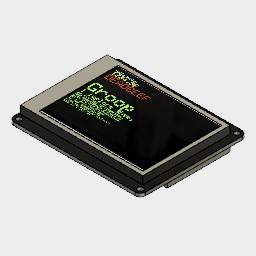
3315  2.4 TFT Feather Wing (Autodesk Fusion 360 design; units mm, degrees)
Autodesk Fusion 360 part; units mm, degrees
note: some values were not read from the file. Set by a fixed rule: which sketch regions a step uses.
sketch "pcb" plane through (0, 0, 0) normal (0, 0, 1) x (1, 0, 0)
  line L0 (0, 0) -> (64.77, 0)
  line L1 (64.77, 0) -> (64.77, 52.578)
  line L2 (64.77, 52.578) -> (0, 52.578)
  line L3 (0, 52.578) -> (0, 0)
  circle A0 centre (2.54, 50.038) radius 1.27
  line L4 (32.385, 52.578) -> (32.385, 0) construction
  line L5 (0, 26.289) -> (64.77, 26.289) construction
  circle A1 centre (62.23, 50.038) radius 1.27
  circle A2 centre (2.54, 2.54) radius 1.27
  circle A3 centre (62.23, 2.54) radius 1.27
  dimension "d1" = 64.77
  dimension "d2" = 52.578
  dimension "d3" = 2.54
  dimension "d4" = 2.54
  dimension "d5" = 2.54
  measures "d1" distance of L1.end L2.end
  measures "d2" distance of L0.start L2.end
  measures "d3" diameter of A0
  measures "d4" distance of L3 A0.centre
  measures "d5" distance of L2 A0.centre
extrude "Extrude1" add sketch "pcb" along normal blind 1.6 makes body 1
fillet "Fillet1" radius 2.54 4 edges at (64.77, 0, 0.8) (0, 0, 0.8) (0, 52.578, 0.8) (64.77, 52.578, 0.8) on bodies 1
sketch "bottom" plane through (0, 0, 0) normal (0, 0, -1) x (1, 0, 0)
  circle A0 centre (62.23, -50.038) radius 1.27
  circle A1 centre (2.54, -2.54) radius 1.27
  circle A2 centre (62.23, -2.54) radius 1.27
  circle A3 centre (2.54, -50.038) radius 1.27
  arc A4 (62.23, -52.578) -> (64.77, -50.038) centre (62.23, -50.038) ccw
  line L0 (64.77, -50.038) -> (64.77, -2.54)
  arc A5 (64.77, -2.54) -> (62.23, 0) centre (62.23, -2.54) ccw
  line L1 (62.23, 0) -> (2.54, 0)
  arc A6 (2.54, 0) -> (0, -2.54) centre (2.54, -2.54) ccw
  line L2 (0, -2.54) -> (0, -50.038)
  arc A7 (0, -50.038) -> (2.54, -52.578) centre (2.54, -50.038) ccw
  line L3 (2.54, -52.578) -> (62.23, -52.578)
  line L4 (62.97, -45.978) -> (57.97, -45.978)
  line L5 (57.97, -45.978) -> (57.97, -14.978)
  line L6 (57.97, -14.978) -> (62.97, -14.978)
  line L7 (62.97, -14.978) -> (62.97, -45.978)
  line L8 (40.17, -45.978) -> (35.17, -45.978)
  line L9 (35.17, -45.978) -> (35.17, -4.978)
  line L10 (35.17, -4.978) -> (40.17, -4.978)
  line L11 (40.17, -4.978) -> (40.17, -45.978)
  line L12 (1.6, -6.8) -> (7.6, -6.8)
  line L13 (7.6, -6.8) -> (7.6, -12.8)
  line L14 (7.6, -12.8) -> (1.6, -12.8)
  line L15 (1.6, -12.8) -> (1.6, -6.8)
  line L16 (1.6, -6.8) -> (7.6, -12.8) construction
  line L17 (7.6, -6.8) -> (1.6, -12.8) construction
  circle A8 centre (4.6, -9.8) radius 1.5
  line L18 (5.5, -17.4) -> (2, -17.4)
  line L19 (2, -17.4) -> (2, -24.4)
  line L20 (2, -24.4) -> (5.5, -24.4)
  line L21 (5.5, -24.4) -> (5.5, -17.4)
  line L22 (15.5, -43.978) -> (0, -43.978)
  line L23 (0, -43.978) -> (0, -29.978)
  line L24 (0, -29.978) -> (15.5, -29.978)
  line L25 (15.5, -29.978) -> (15.5, -43.978)
  point P0 (4.6, -9.8)
  dimension "d9" = 5
  dimension "d10" = 5
  dimension "d11" = 31
  dimension "d12" = 41
  dimension "d13" = 6.6
  dimension "d14" = 6.6
  dimension "d15" = 1.8
  dimension "d16" = 17.8
  dimension "d19" = 6
  dimension "d20" = 6
  dimension "d21" = 6.8
  dimension "d22" = 1.6
  dimension "d23" = 3
  dimension "d28" = 3.5
  dimension "d29" = 7
  dimension "d30" = 2
  dimension "d31" = 17.4
  dimension "d32" = 15.5
  dimension "d33" = 14
  dimension "d34" = 8.6
  measures "d9" distance of L5.end L6.end
  measures "d10" distance of L9.end L10.end
  measures "d11" distance of L4.start L6.end
  measures "d12" distance of L8.start L10.end
  measures "d13" distance of L3 L4
  measures "d14" distance of L3 L8
  measures "d15" distance of L0 L7
  measures "d16" distance of L5 L11
  measures "d19" distance of L13.end L14.end
  measures "d20" distance of L12.end L13.end
  measures "d21" distance of L1 L12
  measures "d22" distance of L2 L15
  measures "d23" diameter of A8
  measures "d28" distance of L18.start L18.end
  measures "d29" distance of L18.start L20.end
  measures "d30" distance of L2 L19
  measures "d31" distance of L1 L18
  measures "d32" distance of L22.start L22.end
  measures "d33" distance of L22.start L24.end
  measures "d34" distance of L3 L22
extrude "Extrude2" add sketch "bottom" along normal blind 3.9 separate body contours L4 L5 L6 L7 | L8 L9 L10 L11 makes body 2 at (61.3033, 25.3113, 0) makes body 3 at (38.5033, 32.3113, 0)
extrude "Extrude3" add sketch "bottom" along normal blind 1.8 separate body contours L12 L13 L14 L15 | A8 makes body 4
extrude "Extrude4" add sketch "bottom" along normal blind 3 separate body contours A8 makes body 5
extrude "Extrude5" add sketch "bottom" along normal blind 1.4 separate body contours L18 L19 L20 L21 makes body 6
extrude "Extrude6" add sketch "bottom" along normal blind 1.7 separate body contours L2 L22 L23 L24 L25 makes body 7
sketch "microSD" plane through (0, 0, -1.7) normal (0, 0, -1) x (1, 0, 0)
  line L0 (15.5, -29.978) -> (0, -29.978)
  line L1 (0, -29.978) -> (0, -43.978)
  line L2 (0, -43.978) -> (15.5, -43.978)
  line L3 (15.5, -43.978) -> (15.5, -29.978)
  circle A0 centre (-8.5, -35.5) radius 11
  dimension "d39" = 22
  measures "d39" diameter of A0
extrude "Extrude7" cut sketch "microSD" against normal blind 1.7 contours L0 L1 A0 picked at (0.2923, -37.9037) bodies 7
sketch "switch" plane through (0, 0, -1.4) normal (0, 0, -1) x (1, 0, 0)
  line L0 (5.5, -24.4) -> (5.5, -17.4)
  line L1 (5.5, -17.4) -> (2, -17.4)
  line L2 (2, -17.4) -> (2, -24.4)
  line L3 (2, -24.4) -> (5.5, -24.4)
  line L4 (2, -20.9) -> (5.5, -20.9)
  line L5 (2, -19.4) -> (3, -19.4)
  line L6 (3, -19.4) -> (3, -22.4)
  line L7 (3, -22.4) -> (2, -22.4)
  line L8 (2, -22.4) -> (2, -19.4)
  line L9 (3, -20.9) -> (2, -20.9) construction
  dimension "d42" = 3
  dimension "d43" = 1
  measures "d42" distance of L5.end L6.end
  measures "d43" distance of L6.end L7.end
extrude "Extrude8" add sketch "switch" along normal blind 1 separate body contours L2 L4 L6 L7 L8 makes body 8
sketch "display" plane through (0, 0, 1.6) normal (0, 0, 1) x (-1, 0, 0)
  arc A0 (-64.77, -50.038) -> (-62.23, -52.578) centre (-62.23, -50.038) ccw
  line L0 (-62.23, -52.578) -> (-2.54, -52.578)
  arc A1 (-2.54, -52.578) -> (0, -50.038) centre (-2.54, -50.038) ccw
  line L1 (0, -50.038) -> (0, -2.54)
  arc A2 (0, -2.54) -> (-2.54, 0) centre (-2.54, -2.54) ccw
  line L2 (-2.54, 0) -> (-62.23, 0)
  arc A3 (-62.23, 0) -> (-64.77, -2.54) centre (-62.23, -2.54) ccw
  line L3 (-64.77, -2.54) -> (-64.77, -50.038)
  circle A4 centre (-62.23, -50.038) radius 1.27
  circle A5 centre (-2.54, -2.54) radius 1.27
  circle A6 centre (-62.23, -2.54) radius 1.27
  circle A7 centre (-2.54, -50.038) radius 1.27
  line L4 (-0.8, -47.778) -> (-61, -47.778)
  line L5 (-61, -47.778) -> (-61, -4.978)
  line L6 (-61, -4.978) -> (-0.8, -4.978)
  line L7 (-0.8, -4.978) -> (-0.8, -47.778)
  dimension "d46" = 60.2
  dimension "d47" = 42.8
  dimension "d48" = 4.8
  dimension "d49" = 0.8
  measures "d46" distance of L4.start L4.end
  measures "d47" distance of L4.start L6.end
  measures "d48" distance of L0 L4
  measures "d49" distance of L1 L7
extrude "Extrude9" add sketch "display" along normal blind 3.9 separate body contours L4 L5 L6 L7 makes body 9
sketch "view" plane through (0, 0, 5.5) normal (0, 0, 1) x (-1, 0, 0)
  line L0 (-0.8, -4.978) -> (-61, -4.978)
  line L1 (-61, -4.978) -> (-61, -47.778)
  line L2 (-61, -47.778) -> (-0.8, -47.778)
  line L3 (-0.8, -47.778) -> (-0.8, -4.978)
  line L4 (-8, -45.778) -> (-59, -45.778)
  line L5 (-59, -45.778) -> (-59, -6.978)
  line L6 (-59, -6.978) -> (-8, -6.978)
  line L7 (-8, -6.978) -> (-8, -45.778)
  dimension "d52" = 2
  dimension "d53" = 2
  dimension "d54" = 2
  dimension "d55" = 7.2
  measures "d52" distance of L0 L6
  measures "d53" distance of L1 L5
  measures "d54" distance of L2 L4
  measures "d55" distance of L3 L7
extrude "Extrude10" cut sketch "view" against normal blind 0.2 contours L4 L5 L6 L7 bodies 9
ref_plane "WorkPlane1" through (30.9, 26.378, 5.7) normal (0, 0, 1) x (1, 0, 0) in component "mount"
sketch "Sketch1" plane through (30.9, 26.378, 5.7) normal (0, 0, 1) x (1, 0, 0) in component "mount"
  line L0 (-32.9, 28.2) -> (35.87, 28.2)
  line L1 (35.87, 28.2) -> (35.87, -28.378)
  line L2 (35.87, -28.378) -> (-32.9, -28.378)
  line L3 (-32.9, -28.378) -> (-32.9, 28.2)
  line L4 (31.33, 26.2) -> (-28.36, 26.2) construction
  line L5 (33.87, -23.838) -> (33.87, 23.66) construction
  line L6 (-30.9, 23.66) -> (-30.9, -23.838) construction
  line L7 (-28.36, -26.378) -> (31.33, -26.378) construction
  line L8 (-22.9, -19.4) -> (28.1, -19.4)
  line L9 (28.1, -19.4) -> (28.1, 19.4)
  line L10 (28.1, 19.4) -> (-22.9, 19.4)
  line L11 (-22.9, 19.4) -> (-22.9, -19.4)
  circle A0 centre (-28.36, -23.838) radius 1.27
  circle A1 centre (31.33, -23.838) radius 1.27
  circle A2 centre (31.33, 23.66) radius 1.27
  circle A3 centre (-28.36, 23.66) radius 1.27
  line L12 (30.1, -21.4) -> (-30.1, -21.4) construction
  line L13 (-30.1, -21.4) -> (-30.1, 21.4) construction
  line L14 (-30.1, 21.4) -> (30.1, 21.4) construction
  line L15 (30.1, 21.4) -> (30.1, -21.4) construction
  circle A4 centre (-28.36, -23.838) radius 2.77
  circle A5 centre (31.33, 23.66) radius 2.77
  circle A6 centre (-28.36, 23.66) radius 2.77
  line L16 (-30.7, -22) -> (-30.7, 22)
  line L17 (-30.7, 22) -> (30.7, 22)
  line L18 (30.7, 22) -> (30.7, -22)
  line L19 (30.7, -22) -> (-30.7, -22)
  circle A7 centre (31.33, -23.838) radius 2.77
  point P0 (30.06, -23.838)
  dimension "d59" = 2
  dimension "d60" = 2
  dimension "d61" = 2
  dimension "d62" = 2
  dimension "d65" = 1.5
  dimension "d66" = 1.5
  dimension "d67" = 1.5
  dimension "d68" = 1.5
  dimension "d74" = 0.6
  measures "d59" distance of L0 L4
  measures "d60" distance of L1 L5
  measures "d61" distance of L3 L6
  measures "d62" distance of L2 L7
extrude "Extrude1'" add sketch "Sketch1" along normal blind 1 separate body contours L0 L1 L2 L3 | A0 | A1 | A2 | A3 | A4 L19 | A4 L19 | A4 A5 A6 L16 L17 L18 L19 A7 | L18 L19 A7 | L18 L19 A7 | A5 L17 L18 | A5 L17 L18 | A6 L17 | A6 L17 makes body 10 in component "mount"
extrude "Extrude2'" add sketch "Sketch1" against normal up to surface (4.1 mm away) contours A0 | A1 | A2 | A3 | A4 L19 | A4 L19 | L18 L19 A7 | L18 L19 A7 | A5 L17 L18 | A5 L17 L18 | A6 L17 | A6 L17 bodies 10 in component "mount"
extrude "Extrude3'" add sketch "Sketch1" against normal blind 6.5 contours A0 | A1 | A2 | A3 bodies 10 in component "mount"
fillet "Fillet1'" radius 2.54 4 edges at (-2, -2, 6.2) (66.77, -2, 6.2) (-2, 54.578, 6.2) (66.77, 54.578, 6.2) on bodies 10 in component "mount"
extrude "Extrude4'" cut sketch "Sketch1" against normal blind 5 contours A4 L19 | A4 A5 A6 L16 L17 L18 L19 A7 | L18 L19 A7 | A5 L17 L18 | A6 L17 picked at (-28.2304, -21.6985) picked at (30.5911, -21.4597) picked at (30.5768, 21.3464) picked at (-27.9175, 21.7429) bodies 10 in component "mount"
sketch "32 holes" plane through (0, 0, -3.9) normal (0, 0, -1) x (1, 0, 0)
  line L0 (40.17, -4.978) -> (35.17, -4.978)
  line L1 (35.17, -4.978) -> (35.17, -45.978)
  line L2 (35.17, -45.978) -> (40.17, -45.978)
  line L3 (40.17, -45.978) -> (40.17, -4.978)
  line L4 (37.67, -4.978) -> (37.67, -45.978) construction
  line L5 (38.94, -45.978) -> (38.94, -4.978) construction
  circle A0 centre (38.94, -44.708) radius 0.635
  circle A1 centre (38.94, -42.168) radius 0.635
  circle A2 centre (38.94, -39.628) radius 0.635
  circle A3 centre (38.94, -37.088) radius 0.635
  circle A4 centre (38.94, -34.548) radius 0.635
  circle A5 centre (38.94, -29.468) radius 0.635
  circle A6 centre (38.94, -26.928) radius 0.635
  circle A7 centre (38.94, -32.008) radius 0.635
  circle A8 centre (38.94, -24.388) radius 0.635
  circle A9 centre (38.94, -21.848) radius 0.635
  circle A10 centre (38.94, -19.308) radius 0.635
  circle A11 centre (38.94, -16.768) radius 0.635
  circle A12 centre (38.94, -14.228) radius 0.635
  circle A13 centre (38.94, -11.688) radius 0.635
  circle A14 centre (38.94, -9.148) radius 0.635
  circle A15 centre (38.94, -6.608) radius 0.635
  circle A16 centre (36.4, -6.608) radius 0.635
  circle A17 centre (36.4, -9.148) radius 0.635
  circle A18 centre (36.4, -11.688) radius 0.635
  circle A19 centre (36.4, -14.228) radius 0.635
  circle A20 centre (36.4, -16.768) radius 0.635
  circle A21 centre (36.4, -19.308) radius 0.635
  circle A22 centre (36.4, -21.848) radius 0.635
  circle A23 centre (36.4, -24.388) radius 0.635
  circle A24 centre (36.4, -26.928) radius 0.635
  circle A25 centre (36.4, -29.468) radius 0.635
  circle A26 centre (36.4, -32.008) radius 0.635
  circle A27 centre (36.4, -34.548) radius 0.635
  circle A28 centre (36.4, -37.088) radius 0.635
  circle A29 centre (36.4, -39.628) radius 0.635
  circle A30 centre (36.4, -42.168) radius 0.635
  circle A31 centre (36.4, -44.708) radius 0.635
  dimension "d101" = 1.27
  dimension "d102" = 1.27
  dimension "d103" = 1.27
  dimension "d104" = 1.27
  dimension "d105" = 1.27
  dimension "d106" = 1.27
  dimension "d107" = 1.27
  dimension "d108" = 2.54
  dimension "d109" = 2.54
  dimension "d110" = 2.54
  dimension "d111" = 2.54
  dimension "d113" = 1.27
  dimension "d114" = 1.27
  dimension "d116" = 1.27
  dimension "d117" = 2.54
  dimension "d118" = 2.54
  dimension "d119" = 2.54
  dimension "d120" = 1.27
  dimension "d121" = 1.27
  dimension "d122" = 1.27
  dimension "d123" = 1.27
  dimension "d124" = 2.54
  dimension "d125" = 2.54
  dimension "d126" = 2.54
  dimension "d127" = 2.54
  dimension "d128" = 1.27
  dimension "d129" = 1.27
  dimension "d130" = 1.27
  dimension "d131" = 2.54
  dimension "d132" = 2.54
  dimension "d133" = 2.54
  dimension "d134" = 1.27
  dimension "d135" = 2.54
  measures "d101" distance of L4 L5
  measures "d102" diameter of A0
  measures "d103" distance of L2 A0.centre
  measures "d104" diameter of A1
  measures "d105" diameter of A2
  measures "d106" diameter of A3
  measures "d107" diameter of A4
  measures "d108" distance of A0.centre A1.centre
  measures "d109" distance of A1.centre A2.centre
  measures "d110" distance of A2.centre A3.centre
  measures "d111" distance of A3.centre A4.centre
  measures "d113" diameter of A5
  measures "d114" diameter of A6
  measures "d116" diameter of A7
  measures "d117" distance of A4.centre A7.centre
  measures "d118" distance of A5.centre A7.centre
  measures "d119" distance of A5.centre A6.centre
  measures "d120" diameter of A8
  measures "d121" diameter of A9
  measures "d122" diameter of A10
  measures "d123" diameter of A11
  measures "d124" distance of A6.centre A8.centre
  measures "d125" distance of A8.centre A9.centre
  measures "d126" distance of A9.centre A10.centre
  measures "d127" distance of A10.centre A11.centre
  measures "d128" diameter of A12
  measures "d129" diameter of A13
  measures "d130" diameter of A14
  measures "d131" distance of A11.centre A12.centre
  measures "d132" distance of A12.centre A13.centre
  measures "d133" distance of A13.centre A14.centre
  measures "d134" diameter of A15
  measures "d135" distance of A14.centre A15.centre
extrude "Extrude12" cut sketch "32 holes" against normal blind 2 contours A0 | A1 | A2 | A3 | A4 | A5 | A6 | A7 | A8 | A9 | A10 | A11 | A12 | A13 | A14 | A15 | A16 | A17 | A18 | A19 | A20 | A21 | A22 | A23 | A24 | A25 | A26 | A27 | A28 | A29 | A30 | A31 bodies 3
sketch "24 holes" plane through (0, 0, -3.9) normal (0, 0, -1) x (1, 0, 0)
  line L0 (62.97, -14.978) -> (57.97, -14.978)
  line L1 (57.97, -14.978) -> (57.97, -45.978)
  line L2 (57.97, -45.978) -> (62.97, -45.978)
  line L3 (62.97, -45.978) -> (62.97, -14.978)
  line L4 (38.94, -45.978) -> (38.94, -4.978)
  line L5 (59.26, -45.978) -> (59.26, -14.978) construction
  circle A0 centre (59.26, -44.708) radius 0.635
  circle A1 centre (59.26, -42.168) radius 0.635
  circle A2 centre (59.26, -39.628) radius 0.635
  circle A3 centre (59.26, -37.088) radius 0.635
  circle A4 centre (59.26, -34.548) radius 0.635
  circle A5 centre (59.26, -32.008) radius 0.635
  circle A6 centre (59.26, -29.468) radius 0.635
  circle A7 centre (59.26, -26.928) radius 0.635
  circle A8 centre (59.26, -24.388) radius 0.635
  circle A9 centre (59.26, -21.848) radius 0.635
  circle A10 centre (59.26, -19.308) radius 0.635
  circle A11 centre (59.26, -16.768) radius 0.635
  line L6 (60.47, -14.978) -> (60.47, -45.978) construction
  circle A12 centre (61.68, -16.768) radius 0.635
  circle A13 centre (61.68, -19.308) radius 0.635
  circle A14 centre (61.68, -21.848) radius 0.635
  circle A15 centre (61.68, -24.388) radius 0.635
  circle A16 centre (61.68, -26.928) radius 0.635
  circle A17 centre (61.68, -29.468) radius 0.635
  circle A18 centre (61.68, -32.008) radius 0.635
  circle A19 centre (61.68, -34.548) radius 0.635
  circle A20 centre (61.68, -37.088) radius 0.635
  circle A21 centre (61.68, -39.628) radius 0.635
  circle A22 centre (61.68, -42.168) radius 0.635
  circle A23 centre (61.68, -44.708) radius 0.635
  dimension "d141" = 20.32
  dimension "d142" = 1.27
  dimension "d143" = 1.27
  dimension "d144" = 1.27
  dimension "d145" = 1.27
  dimension "d146" = 2.54
  dimension "d147" = 2.54
  dimension "d148" = 1.27
  dimension "d149" = 1.27
  dimension "d150" = 1.27
  dimension "d151" = 2.54
  dimension "d152" = 2.54
  dimension "d153" = 2.54
  dimension "d154" = 1.27
  dimension "d155" = 1.27
  dimension "d156" = 1.27
  dimension "d157" = 2.54
  dimension "d158" = 2.54
  dimension "d160" = 2.54
  dimension "d161" = 1.27
  dimension "d162" = 1.27
  dimension "d163" = 1.27
  dimension "d164" = 2.54
  dimension "d165" = 2.54
  dimension "d166" = 2.54
  measures "d141" distance of L4 L5
  measures "d142" diameter of A0
  measures "d143" diameter of A1
  measures "d144" diameter of A2
  measures "d145" distance of L2 A0.centre
  measures "d146" distance of A0.centre A1.centre
  measures "d147" distance of A1.centre A2.centre
  measures "d148" diameter of A3
  measures "d149" diameter of A4
  measures "d150" diameter of A5
  measures "d151" distance of A2.centre A3.centre
  measures "d152" distance of A3.centre A4.centre
  measures "d153" distance of A4.centre A5.centre
  measures "d154" diameter of A6
  measures "d155" diameter of A7
  measures "d156" diameter of A8
  measures "d157" distance of A5.centre A6.centre
  measures "d158" distance of A6.centre A7.centre
  measures "d160" distance of A7.centre A8.centre
  measures "d161" diameter of A9
  measures "d162" diameter of A10
  measures "d163" diameter of A11
  measures "d164" distance of A8.centre A9.centre
  measures "d165" distance of A9.centre A10.centre
  measures "d166" distance of A10.centre A11.centre
extrude "Extrude13" cut sketch "24 holes" against normal blind 2 contours A0 | A1 | A2 | A3 | A4 | A5 | A6 | A7 | A8 | A9 | A10 | A11 | A12 | A13 | A14 | A15 | A16 | A17 | A18 | A19 | A20 | A21 | A22 | A23 bodies 2
sketch "Solder Pads" plane through (0, 0, 0) normal (0, 0, 1) x (1, 0, 0)
  line L0 (2.54, 0) -> (62.23, 0)
  line L1 (62.23, 52.578) -> (2.54, 52.578)
  line L2 (42.75, 0) -> (42.75, 52.578) construction
  line L3 (54.815, 52.578) -> (54.815, 0) construction
  circle A0 centre (42.75, 44.708) radius 0.635
  circle A1 centre (42.75, 42.168) radius 0.635
  circle A2 centre (42.75, 39.628) radius 0.635
  circle A3 centre (42.75, 37.088) radius 0.635
  circle A4 centre (42.75, 34.548) radius 0.635
  circle A5 centre (42.75, 32.008) radius 0.635
  circle A6 centre (42.75, 29.468) radius 0.635
  circle A7 centre (42.75, 26.928) radius 0.635
  circle A8 centre (42.75, 24.388) radius 0.635
  circle A9 centre (42.75, 21.848) radius 0.635
  circle A10 centre (42.75, 19.308) radius 0.635
  circle A11 centre (42.75, 16.768) radius 0.635
  circle A12 centre (42.75, 14.228) radius 0.635
  circle A13 centre (42.75, 11.688) radius 0.635
  circle A14 centre (42.75, 9.148) radius 0.635
  circle A15 centre (42.75, 6.608) radius 0.635
  circle A16 centre (54.815, 44.708) radius 0.635
  circle A17 centre (54.815, 42.168) radius 0.635
  circle A18 centre (54.815, 29.468) radius 0.635
  circle A19 centre (54.815, 26.928) radius 0.635
  circle A20 centre (54.815, 24.388) radius 0.635
  circle A21 centre (54.815, 21.848) radius 0.635
  circle A22 centre (54.815, 19.308) radius 0.635
  circle A23 centre (54.815, 16.768) radius 0.635
  circle A24 centre (29.21, 43.942) radius 0.635
  line L4 (32.385, 52.578) -> (32.385, 0)
  circle A25 centre (20.32, 43.942) radius 0.635
  circle A26 centre (17.145, 43.942) radius 0.635
  dimension "d171" = 1.27
  dimension "d173" = 1.27
  dimension "d174" = 1.27
  dimension "d175" = 1.27
  dimension "d176" = 2.54
  dimension "d177" = 2.54
  dimension "d178" = 2.54
  dimension "d179" = 1.27
  dimension "d180" = 1.27
  dimension "d181" = 1.27
  dimension "d182" = 1.27
  dimension "d183" = 1.27
  dimension "d184" = 1.27
  dimension "d185" = 2.54
  dimension "d186" = 2.54
  dimension "d187" = 2.54
  dimension "d188" = 2.54
  dimension "d189" = 2.54
  dimension "d190" = 2.54
  dimension "d191" = 1.27
  dimension "d192" = 1.27
  dimension "d193" = 1.27
  dimension "d194" = 1.27
  dimension "d195" = 1.27
  dimension "d196" = 1.27
  dimension "d197" = 2.54
  dimension "d198" = 2.54
  dimension "d199" = 2.54
  dimension "d200" = 2.54
  dimension "d201" = 2.54
  dimension "d202" = 2.54
  dimension "d203" = 1.27
  dimension "d205" = 1.27
  dimension "d206" = 1.27
  dimension "d207" = 2.54
  dimension "d208" = 12.7
  dimension "d209" = 1.27
  dimension "d210" = 1.27
  dimension "d211" = 1.27
  dimension "d212" = 1.27
  dimension "d213" = 1.27
  dimension "d214" = 2.54
  dimension "d215" = 2.54
  dimension "d216" = 2.54
  dimension "d217" = 2.54
  dimension "d218" = 2.54
  dimension "d219" = 1.27
  dimension "d221" = 3.175
  dimension "d222" = 1.27
  dimension "d223" = 1.27
  dimension "d226" = 8.89
  dimension "d227" = 3.175
  measures "d171" diameter of A0
  measures "d173" diameter of A1
  measures "d174" diameter of A2
  measures "d175" diameter of A3
  measures "d176" distance of A0.centre A1.centre
  measures "d177" distance of A1.centre A2.centre
  measures "d178" distance of A2.centre A3.centre
  measures "d179" diameter of A4
  measures "d180" diameter of A5
  measures "d181" diameter of A6
  measures "d182" diameter of A7
  measures "d183" diameter of A8
  measures "d184" diameter of A9
  measures "d185" distance of A3.centre A4.centre
  measures "d186" distance of A4.centre A5.centre
  measures "d187" distance of A5.centre A6.centre
  measures "d188" distance of A6.centre A7.centre
  measures "d189" distance of A7.centre A8.centre
  measures "d190" distance of A8.centre A9.centre
  measures "d191" diameter of A10
  measures "d192" diameter of A11
  measures "d193" diameter of A12
  measures "d194" diameter of A13
  measures "d195" diameter of A14
  measures "d196" diameter of A15
  measures "d197" distance of A9.centre A10.centre
  measures "d198" distance of A10.centre A11.centre
  measures "d199" distance of A11.centre A12.centre
  measures "d200" distance of A12.centre A13.centre
  measures "d201" distance of A13.centre A14.centre
  measures "d202" distance of A14.centre A15.centre
  measures "d203" diameter of A16
  measures "d205" diameter of A17
  measures "d206" diameter of A18
  measures "d207" distance of A16.centre A17.centre
  measures "d208" distance of A17.centre A18.centre
  measures "d209" diameter of A19
  measures "d210" diameter of A20
  measures "d211" diameter of A21
  measures "d212" diameter of A22
  measures "d213" diameter of A23
  measures "d214" distance of A18.centre A19.centre
  measures "d215" distance of A19.centre A20.centre
  measures "d216" distance of A20.centre A21.centre
  measures "d217" distance of A21.centre A22.centre
  measures "d218" distance of A22.centre A23.centre
  measures "d219" diameter of A24
  measures "d221" distance of A24.centre L4
  measures "d222" diameter of A25
  measures "d223" diameter of A26
  measures "d226" distance of A24.centre A25.centre
  measures "d227" distance of A25.centre A26.centre
component "mount" placed x (1, 0, 0) y (0, 1, 0) z (0, 0, 1) at (0, 0, 0)
equation "HoleDia = 1.27 mm"
equation "HoleSpace = 0.1 in"
equation "d101 = HoleSpace / 2"
equation "d102 = HoleDia"
equation "d103 = HoleSpace / 2"
equation "d104 = HoleDia"
equation "d105 = HoleDia"
equation "d106 = HoleDia"
equation "d107 = HoleDia"
equation "d108 = HoleSpace"
equation "d109 = HoleSpace"
equation "d110 = HoleSpace"
equation "d111 = HoleSpace"
equation "d113 = HoleDia"
equation "d114 = HoleDia"
equation "d116 = HoleDia"
equation "d117 = HoleSpace"
equation "d118 = HoleSpace"
equation "d119 = HoleSpace"
equation "d120 = HoleDia"
equation "d121 = HoleDia"
equation "d122 = HoleDia"
equation "d123 = HoleDia"
equation "d124 = HoleSpace"
equation "d125 = HoleSpace"
equation "d126 = HoleSpace"
equation "d127 = HoleSpace"
equation "d128 = HoleDia"
equation "d129 = HoleDia"
equation "d130 = HoleDia"
equation "d131 = HoleSpace"
equation "d132 = HoleSpace"
equation "d133 = HoleSpace"
equation "d134 = HoleDia"
equation "d135 = HoleSpace"
equation "HoleDepth = 2 mm"
equation "d137 = -HoleDepth"
equation "d142 = HoleDia"
equation "d143 = HoleDia"
equation "d144 = HoleDia"
equation "d145 = HoleSpace / 2"
equation "d146 = HoleSpace"
equation "d147 = HoleSpace"
equation "d148 = HoleDia"
equation "d149 = HoleDia"
equation "d150 = HoleDia"
equation "d151 = HoleSpace"
equation "d152 = HoleSpace"
equation "d153 = HoleSpace"
equation "d154 = HoleDia"
equation "d155 = HoleDia"
equation "d156 = HoleDia"
equation "d157 = HoleSpace"
equation "d158 = HoleSpace"
equation "d160 = HoleSpace"
equation "d161 = HoleDia"
equation "d162 = HoleDia"
equation "d163 = HoleDia"
equation "d164 = HoleSpace"
equation "d165 = HoleSpace"
equation "d166 = HoleSpace"
equation "d167 = -HoleDepth"
equation "d171 = HoleDia"
equation "d173 = HoleDia"
equation "d174 = HoleDia"
equation "d175 = HoleDia"
equation "d176 = HoleSpace"
equation "d177 = HoleSpace"
equation "d178 = HoleSpace"
equation "d179 = HoleDia"
equation "d180 = HoleDia"
equation "d181 = HoleDia"
equation "d182 = HoleDia"
equation "d183 = HoleDia"
equation "d184 = HoleDia"
equation "d185 = HoleSpace"
equation "d186 = HoleSpace"
equation "d187 = HoleSpace"
equation "d188 = HoleSpace"
equation "d189 = HoleSpace"
equation "d190 = HoleSpace"
equation "d191 = HoleDia"
equation "d192 = HoleDia"
equation "d193 = HoleDia"
equation "d194 = HoleDia"
equation "d195 = HoleDia"
equation "d196 = HoleDia"
equation "d197 = HoleSpace"
equation "d198 = HoleSpace"
equation "d199 = HoleSpace"
equation "d200 = HoleSpace"
equation "d201 = HoleSpace"
equation "d202 = HoleSpace"
equation "d203 = HoleDia"
equation "d205 = HoleDia"
equation "d206 = HoleDia"
equation "d207 = HoleSpace"
equation "d208 = HoleSpace * 5"
equation "d209 = HoleDia"
equation "d210 = HoleDia"
equation "d211 = HoleDia"
equation "d212 = HoleDia"
equation "d213 = HoleDia"
equation "d214 = HoleSpace"
equation "d215 = HoleSpace"
equation "d216 = HoleSpace"
equation "d217 = HoleSpace"
equation "d218 = HoleSpace"
equation "d219 = HoleDia"
equation "d222 = HoleDia"
equation "d223 = HoleDia"
named bodies: "pcb", "header medium", "header long", "button base", "microSD", "switch base", "display", "button", "switch"
